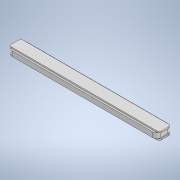
# Autodesk Inventor part: GT2Rack
Saved by Autodesk Inventor 2022 (Build 260153000, 153)
## iProperties
Created: 2022-08-08
Part Number: GT2Rack
Material: Genérico
Document SubType Name: Modeling
Designer: JK
Density: 1 g/cm^3
Appearance: Valor por defecto
Author: JK
Autodesk Inventor part; units mm, degrees
ref_plane "YZ Plane" through (0, 0, 0) normal (1, 0, 0) x (0, 1, 0)
ref_plane "XZ Plane" through (0, 0, 0) normal (0, 1, 0) x (-1, 0, 0)
ref_plane "XY Plane" through (0, 0, 0) normal (0, 0, 1) x (1, 0, 0)
sketch "Boceto1" plane through (0, 0, 0) normal (0, 1, 0) x (-1, 0, 0)
  line L0 (96, 7.5) -> (-96, 7.5)
  line L1 (-96, 7.5) -> (-96, -7.5)
  line L2 (-96, -7.5) -> (96, -7.5)
  line L3 (96, -7.5) -> (96, 7.5)
  line L4 (96, 7.5) -> (-96, -7.5) construction
  line L5 (-96, 7.5) -> (96, -7.5) construction
  point P0 (0, 0)
  dimension "d0" = 192
  dimension "d1" = 15
  constraints: 12 end point, 2 midpoint, 2 parallel, 1 horizontal, 1 perpendicular
  measures "d0" distance between parallel lines of L3 L1
  measures "d1" distance of L2.end L0.start
extrude "Extrusión1" add sketch "Boceto1" along normal blind 10
sketch "Boceto2" plane through (0, 0, 0) normal (1, 0, 0) x (0, 1, 0)
  line L0 (0, 7.5) -> (10, 7.5) projected
  line L1 (1.75, 7.5) -> (8.25, 7.5)
  line L2 (8.25, 7.5) -> (8.25, 9.5)
  line L3 (8.25, 9.5) -> (1.75, 9.5)
  line L4 (1.75, 9.5) -> (1.75, 7.5)
  line L5 (0, -7.5) -> (0, 7.5) projected
  line L6 (0, -7.5) -> (10, -7.5) projected
  line L7 (1.75, -7.5) -> (8.25, -7.5)
  line L8 (8.25, -7.5) -> (8.25, -9.5)
  line L9 (8.25, -9.5) -> (1.75, -9.5)
  line L10 (1.75, -9.5) -> (1.75, -7.5)
  point P0 (0, 0)
  dimension "d4" = 6.5
  dimension "d5" = 1.75
  dimension "d6" = 2
  constraints: 16 end point, 4 parallel, 3 collinear, 2 horizontal, 2 perpendicular, 2 point on line
  measures "d4" distance between parallel lines of L4 L2
  measures "d5" distance between parallel lines of L5 L4
  measures "d6" distance between parallel lines of L0 L3
extrude "Extrusión2" add sketch "Boceto2" along normal mid plane 192
sketch "Boceto4" plane through (-96, 0, -7.5) normal (-1, 0, 0) x (0, 0, 1)
  line L0 (15, 1.75) -> (17, 1.75) projected
  line L1 (0, 8.25) -> (-2, 8.25) projected
  line L2 (17, 1.75) -> (-2, 1.75)
  line L3 (-2, 1.75) -> (-2, 8.25)
  line L4 (-2, 8.25) -> (17, 8.25)
  line L5 (17, 8.25) -> (17, 1.75)
  point P0 (7.5, 0)
  point P1 (15, 1.75)
  point P2 (0, 8.25)
  constraints: 8 end point, 2 parallel, 1 horizontal, 1 perpendicular
extrude "Extrusión3" cut sketch "Boceto4" against normal blind 1
sketch "Boceto5" plane through (96, 0, 7.5) normal (1, 0, 0) x (0, 0, -1)
  line L0 (0, 8.25) -> (-2, 8.25) projected
  line L1 (17, 1.75) -> (17, 8.25) projected
  line L2 (-2, 8.25) -> (17, 8.25)
  line L3 (17, 8.25) -> (17, 1.75)
  line L4 (17, 1.75) -> (-2, 1.75)
  line L5 (-2, 1.75) -> (-2, 8.25)
  point P0 (7.5, 0)
  point P1 (17, 8.25)
  point P2 (0, 8.25)
  constraints: 8 end point, 2 parallel, 1 horizontal, 1 perpendicular
extrude "Extrusión4" cut sketch "Boceto5" against normal blind 1
fillet "Empalme1" radius 5 4 edges at (95, 5, -9.5) (95, 5, 9.5) (-95, 5, -9.5) (-95, 5, 9.5)
fillet "Empalme2" radius 3 8 edges at (96, 9.125, 7.5) (96, 0.875, 7.5) (96, 9.125, -7.5) (96, 0.875, -7.5) (-96, 0.875, 7.5) (-96, 9.125, 7.5) (-96, 0.875, -7.5) (-96, 9.125, -7.5)
